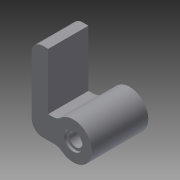
# Autodesk Inventor part: goal holder
Saved by Autodesk Inventor 2015 (Build 190159000, 159)
## iProperties
Created: 2014-11-06
Part Number: goal holder
Material: Generic
Document SubType Name: Modeling
Designer: jesse
Density: 1 g/cm^3
Appearance: Default
Author: jesse
Autodesk Inventor part; units mm, degrees
ref_plane "YZ Plane" through (0, 0, 0) normal (1, 0, 0) x (0, 1, 0)
ref_plane "XZ Plane" through (0, 0, 0) normal (0, 1, 0) x (-1, 0, 0)
ref_plane "XY Plane" through (0, 0, 0) normal (0, 0, 1) x (1, 0, 0)
sketch "Sketch1" plane through (0, 0, 0) normal (0, 0, 1) x (1, 0, 0)
  circle A0 centre (0, 0) radius 11 projected
  circle A1 centre (0, 0) radius 1.75 projected
  circle A2 centre (-8, 0) radius 1.75 projected
  circle A3 centre (0, 8) radius 1.75 projected
  circle A4 centre (8, 0) radius 1.75 projected
  circle A5 centre (0, -8) radius 1.75 projected
extrude "Extrusion1" add sketch "Sketch1" along normal blind 9.525
sketch "Sketch2" plane through (0, 0, 9.525) normal (0, 0, 1) x (1, 0, 0)
  circle A0 centre (0, 0) radius 11 projected
  line L0 (9.0377, 6.2705) -> (14.8574, 6.2705)
  line L1 (14.8574, 6.2705) -> (14.8574, 19.7717)
  line L2 (22.8575, 39.6603) -> (24.5877, 39.6603)
  line L3 (24.5877, 39.6603) -> (24.5877, -7.2164)
  line L4 (24.5877, -7.2164) -> (8.302, -7.2164)
  line L5 (22.8575, 39.6603) -> (14.8574, 39.6603)
  line L6 (14.8574, 19.7717) -> (14.8574, 39.6603)
  point P0 (-11, -11)
  dimension "d11" = 46.8767
  dimension "d12" = 13.4869
  constraints: 14 end point, 3 perpendicular, 2 point on circle, 1 horizontal, 1 parallel, 1 vertical
  measures "d11" distance of L2.end L3.end
  measures "d12" distance between parallel lines of L0 L4
extrude "Extrusion2" add sketch "Sketch2" along normal blind 23.8125
mirror "Mirror1" about plane through (0, 0, 0) normal (1, 0, 0) remove original yes
sketch "Sketch3" plane through (-24.5877, -7.2164, 33.3375) normal (0, 0, 1) x (1, 0, 0)
  circle A0 centre (24.5877, 7.2164) radius 3.9688
  dimension "d4" = 7.9375
  constraints: 1 centre point, 1 coincident
  measures "d4" diameter of A0
extrude "Extrusion3" cut sketch "Sketch3" against normal blind 12.4
sketch "Sketch4" plane through (-24.5877, -7.2164, 33.3375) normal (0, 0, 1) x (1, 0, 0)
  circle A0 centre (24.5877, 7.2164) radius 5.5
  dimension "d7" = 11
  constraints: 1 centre point, 1 coincident
  measures "d7" diameter of A0
extrude "Extrusion4" cut sketch "Sketch4" against normal blind 1.5
fillet "Fillet1" radius 6.35 4 edges at (-24.5877, -7.2164, 21.4312) (-8.302, -7.2164, 21.4312) (-9.0377, 6.2705, 21.4312) (-24.5877, 39.6603, 21.4312)
body "Solid1"
